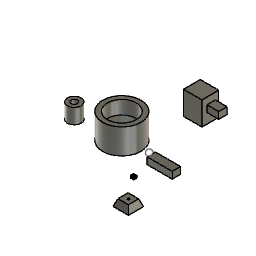
Week 2 Class (Autodesk Fusion 360 design; units mm, degrees)
Autodesk Fusion 360 part; units mm, degrees
sketch "Sketch1" plane through (0, 0, 0) normal (0, 0, 1) x (1, 0, 0)
  line L0 (0, 0) -> (55, 0)
  line L1 (55, 0) -> (55, 50)
  line L2 (55, 50) -> (0, 50)
  line L3 (0, 50) -> (0, 0)
  constraint horizontal L0
  constraint vertical L1
  constraint horizontal L2
  constraint vertical L3
  constraint coincident L0.start L3.end
extrude "Extrude1" add sketch "Sketch1" along normal blind 70 makes body 1
sketch "Sketch2" plane through (55, 0, 0) normal (1, 0, 0) x (0, 1, 0)
  line L0 (0, 0) -> (50, 0)
  line L1 (50, 0) -> (50, 70)
  line L2 (50, 70) -> (0, 70)
  line L3 (0, 70) -> (0, 0)
  line L4 (15, 50) -> (40, 50)
  line L5 (40, 50) -> (40, 30)
  line L6 (40, 30) -> (15, 30)
  line L7 (15, 30) -> (15, 50)
  constraint horizontal L4
  constraint vertical L5
  constraint horizontal L6
  constraint vertical L7
extrude "Extrude2" add sketch "Sketch2" along normal blind 35 contours L4 L5 L6 L7 bodies 1
sketch "Sketch3" plane through (0, 0, 0) normal (0, -1, 0) x (1, 0, 0)
  line L0 (0, 0) -> (55, 0)
  line L1 (55, 0) -> (55, 70)
  line L2 (55, 70) -> (0, 70)
  line L3 (0, 70) -> (0, 0)
sketch "Sketch4" plane through (0, 0, 0) normal (0, 1, 0) x (1, 0, 0)
sketch "Sketch5" plane through (0, 0, 0) normal (0, 1, 0) x (1, 0, 0)
move_body "Move1" bodies 1 to x (1, 0, 0) y (0, 1, 0) z (0, 0, 1) at (0, 35, 0)
sketch "Sketch6" plane through (0, 0, 0) normal (0, 0, 1) x (1, 0, 0)
  circle A0 centre (0, 0) radius 20.4411
  constraint coincident A0.centre origin
extrude "Extrude3" add sketch "Sketch6" along normal blind 45 separate body makes body 2
move_body "Move2" bodies 2 to x (1, 0, 0) y (0, 1, 0) z (0, 0, 1) at (-3.3511, -40.3603, -9.1078)
sketch "Sketch7" plane through (0, 0, 35.8922) normal (0, 0, 1) x (-1, 0, 0)
  circle A0 centre (3.3511, 40.3603) radius 20.4411
  circle A1 centre (3.3511, 40.3603) radius 9.1882
  dimension "d7" = 18.3763
  constraint concentric A0 A1
  measures "d7" diameter of A1
extrude "Extrude4" cut sketch "Sketch7" against normal blind 25 contours A1 bodies 2
extrude "Extrude5" cut 1 faces at (-2.352, -37.8976, 10.8922) along direction (0, 0, -1) blind 129 on bodies 2 bodies 2
move_body "Move3" bodies 2 to x (1, 0, 0) y (0, 1, 0) z (0, 0, 1) at (3.9091, 37.2212, 0)
sketch "Sketch8" plane through (0, 0, 0) normal (1, 0, 0) x (0, 1, 0)
sketch "Sketch9" plane through (0, 0, 0) normal (0, 0, 1) x (1, 0, 0)
sketch "Sketch10" plane through (0, 0, 0) normal (0, 0, 1) x (1, 0, 0)
move_body "Move4" bodies 2 to x (1, 0, 0) y (0, 1, 0) z (0, 0, 1) at (-134.413, -4.3083, 34.1078)
move_body "Move5" bodies 1 to x (1, 0, 0) y (0, 1, 0) z (0, 0, 1) at (64.4102, 84.3152, 34.3939)
sketch "Sketch11" plane through (0, 0, 0) normal (0, 0, 1) x (1, 0, 0)
  circle A0 centre (0, 0) radius 57.0088
  constraint coincident A0.centre origin
extrude "Extrude6" add sketch "Sketch11" along normal blind 75 separate body makes body 3
sketch "Sketch12" plane through (0, 0, 0) normal (0, 0, 1) x (1, 0, 0)
sketch "Sketch13" plane through (0, 0, 75) normal (0, 0, 1) x (-1, 0, 0)
  circle A0 centre (0, 0) radius 57.0088
  circle A1 centre (0, 0) radius 43.0116
  constraint concentric A0 A1
extrude "Extrude7" cut sketch "Sketch13" against normal blind 40 contours A1 bodies 3
sketch "Sketch14" plane through (0, 0, 35) normal (0, 0, 1) x (-1, 0, 0)
  circle A0 centre (0, 0) radius 43.0116
  circle A1 centre (0, 0) radius 11.2283
  constraint coincident A0.centre A1.centre
extrude "Extrude8" cut sketch "Sketch14" against normal blind 90 contours A1 bodies 3
form "Form1" [no effect]
sketch "Sketch15" plane through (0, 0, 0) normal (0, 0, 1) x (1, 0, 0)
  line L0 (100, 0) -> (175, 0)
  line L1 (175, 0) -> (175, -25)
  line L2 (175, -25) -> (100, -25)
  line L3 (100, -25) -> (100, 0)
  constraint horizontal L0
  constraint vertical L1
  constraint horizontal L2
  constraint vertical L3
extrude "Extrude9" add sketch "Sketch15" along normal blind 20 separate body makes body 4
sketch "Sketch16" plane through (0, 0, 20) normal (0, 0, 1) x (-1, 0, 0)
  line L0 (-100, 25) -> (-175, 25)
  line L1 (-175, 25) -> (-175, 0)
  line L2 (-175, 0) -> (-100, 0)
  line L3 (-100, 0) -> (-100, 25)
  line L4 (-58.674, 80.0041, -18.6782) -> (-104.674, 80.0041, -18.6782)
  line L5 (-104.674, 80.0041, -18.6782) -> (-104.674, 125.0041, -18.6782)
  line L6 (-104.674, 125.0041, -18.6782) -> (-58.674, 125.0041, -18.6782)
  line L7 (-58.674, 125.0041, -18.6782) -> (-58.674, 80.0041, -18.6782)
extrude "Extrude10" add sketch "Sketch16" along normal blind 20 draft -20 separate body contours L4 L5 L6 L7 in plane through (0, 0, 1.3218) normal (0, 0, 1) makes body 5
move_face "MoveFace1" by (70, -50, 0) 1 faces at (86.9142, -97.4306, 21.3218) on bodies 5
move_body "Move6" bodies 5 to x (1, 0, 0) y (0, 1, 0) z (0, 0, 1) at (100, -60, 0)
move_body "Move7" bodies 2 to x (1, 0, 0) y (0, 1, 0) z (0, 0, 1) at (1.9174, -2.3531, -31.6058)
sketch "Sketch17" plane through (0, 0, 21.3218) normal (0, 0, 1) x (-1, 0, 0)
  line L0 (-165.9534, 147.2836) -> (-165.9534, 177.7247)
  line L1 (-165.9534, 177.7247) -> (-197.3946, 177.7247)
  line L2 (-197.3946, 177.7247) -> (-197.3946, 147.2836)
  line L3 (-197.3946, 147.2836) -> (-165.9534, 147.2836)
  line L4 (-180, 160) -> (-185, 160)
  line L5 (-185, 160) -> (-185, 165)
  line L6 (-185, 165) -> (-180, 165)
  line L7 (-180, 165) -> (-180, 160)
  constraint horizontal L4
  constraint vertical L5
  constraint horizontal L6
  constraint vertical L7
extrude "Extrude11" cut sketch "Sketch17" against normal blind 110 contours L4 L5 L6 L7 bodies 5
sketch "Sketch18" plane through (0, 0, 0) normal (0, 0, 1) x (1, 0, 0)
  spline S0 degree 3 poles (74.8233, 9.1575) (74.7545, 9.3692) (74.5561, 9.5253) (74.3206, 9.5253) knots 0 0 0 0 1 1 1 1
  line L0 (74.3206, 9.5253) -> (74.056, 9.5253)
  line L1 (74.056, 9.5253) -> (74.056, 10.319)
  arc A0 (73.7914, 10.5836) -> (74.056, 10.319) centre (73.7914, 10.319) cw
  line L2 (73.7914, 10.5836) -> (72.2039, 10.5836)
  line L3 (72.2039, 10.5836) -> (72.2039, 11.1128)
  line L4 (72.2039, 11.1128) -> (72.7331, 11.1128)
  arc A1 (72.9977, 11.3774) -> (72.7331, 11.1128) centre (72.7331, 11.3774) cw
  line L5 (72.9977, 11.3774) -> (72.9977, 11.9065)
  line L6 (72.9977, 11.9065) -> (73.5268, 11.9065)
  arc A2 (74.056, 12.4357) -> (73.5268, 11.9065) centre (73.5268, 12.4357) cw
  line L7 (74.056, 12.4357) -> (74.056, 12.5442)
  spline S1 degree 3 poles (74.056, 12.5442) (74.8312, 12.232) (75.3789, 11.4726) (75.3789, 10.5836) knots 0 0 0 0 1 1 1 1
  spline S2 degree 3 poles (75.3789, 10.5836) (75.3789, 10.0333) (75.1673, 9.5332) (74.8233, 9.1575) knots 0 0 0 0 1 1 1 1
  spline S3 degree 3 poles (72.9977, 8.4855) (71.9526, 8.6151) (71.1456, 9.5041) (71.1456, 10.5836) knots 0 0 0 0 1 1 1 1
  spline S4 degree 3 poles (71.1456, 10.5836) (71.1456, 10.7477) (71.1668, 10.9064) (71.2011, 11.0572) knots 0 0 0 0 1 1 1 1
  line L8 (71.2011, 11.0572) -> (72.4685, 9.7899)
  line L9 (72.4685, 9.7899) -> (72.4685, 9.5253)
  arc A3 (72.9977, 8.9961) -> (72.4685, 9.5253) centre (72.9977, 9.5253) cw
  arc A4 (70.6164, 10.5836) -> (73.2623, 13.2295) centre (73.2623, 10.5836) cw
  arc A5 (73.2623, 7.9378) -> (70.6164, 10.5836) centre (73.2623, 10.5836) cw
  arc A6 (75.9081, 10.5836) -> (73.2623, 7.9378) centre (73.2623, 10.5836) cw
  arc A7 (73.2623, 13.2295) -> (75.9081, 10.5836) centre (73.2623, 10.5836) cw
sketch "Sketch19" plane through (0, 0, 0) normal (0, 0, 1) x (1, 0, 0)
  line L0 (73, 9) -> (73, 8.5)
  constraint vertical L0
sketch "Sketch20" plane through (0, 0, 0) normal (0, 0, 1) x (1, 0, 0)
sketch "Sketch21" plane through (0, 0, 0) normal (0, 0, 1) x (1, 0, 0)
sketch "Sketch22" plane through (0, 0, 0) normal (0, 0, 1) x (1, 0, 0)
sketch "Sketch23" plane through (0, 0, 0) normal (0, 0, 1) x (1, 0, 0)
  line L0 (120, -85) -> (110, -85)
  line L1 (110, -85) -> (110, -75)
  line L2 (110, -75) -> (120, -75)
  line L3 (120, -75) -> (120, -85)
  line L4 (120, -85) -> (110, -75) construction
  line L5 (110, -85) -> (120, -75) construction
  line L6 (117, -82) -> (113, -82)
  line L7 (113, -82) -> (113, -78)
  line L8 (113, -78) -> (117, -78)
  line L9 (117, -78) -> (117, -82)
  line L10 (117, -82) -> (113, -78) construction
  line L11 (113, -82) -> (117, -78) construction
  line L12 (110, -75) -> (113.5, -75)
  line L13 (113.5, -75) -> (113.5, -78.5)
  line L14 (113.5, -78.5) -> (110, -78.5)
  line L15 (110, -78.5) -> (110, -75)
  line L16 (120, -75) -> (116.5, -75)
  line L17 (116.5, -75) -> (116.5, -78.5)
  line L18 (116.5, -78.5) -> (120, -78.5)
  line L19 (120, -78.5) -> (120, -75)
  line L20 (110, -85) -> (113.5, -85)
  line L21 (113.5, -85) -> (113.5, -81.5)
  line L22 (113.5, -81.5) -> (110, -81.5)
  line L23 (110, -81.5) -> (110, -85)
  line L24 (120, -85) -> (116.5, -85)
  line L25 (116.5, -85) -> (116.5, -81.5)
  line L26 (116.5, -81.5) -> (120, -81.5)
  line L27 (120, -81.5) -> (120, -85)
  line L28 (113.5, -78.5) -> (111, -78.5)
  line L29 (111, -78.5) -> (111, -76)
  line L30 (111, -76) -> (113.5, -76)
  line L31 (113.5, -76) -> (113.5, -78.5)
  line L32 (116.5, -78.5) -> (119, -78.5)
  line L33 (119, -78.5) -> (119, -76)
  line L34 (119, -76) -> (116.5, -76)
  line L35 (116.5, -76) -> (116.5, -78.5)
  line L36 (116.5, -81.5) -> (119, -81.5)
  line L37 (119, -81.5) -> (119, -84)
  line L38 (119, -84) -> (116.5, -84)
  line L39 (116.5, -84) -> (116.5, -81.5)
  line L40 (113.5, -81.5) -> (111, -81.5)
  line L41 (111, -81.5) -> (111, -84)
  line L42 (111, -84) -> (113.5, -84)
  line L43 (113.5, -84) -> (113.5, -81.5)
  line L44 (113, -78) -> (114, -78)
  line L45 (117, -78) -> (116, -78)
  line L46 (113, -78) -> (113, -79)
  line L47 (113, -82) -> (113, -81)
  line L48 (113, -82) -> (114, -82)
  line L49 (117, -82) -> (117, -81)
  line L50 (117, -82) -> (116, -82)
  line L51 (114, -78) -> (112, -76)
  line L52 (114, -78) -> (116.8284, -78) construction
  line L53 (113, -79) -> (111, -77)
  line L54 (113, -79) -> (115.8284, -79) construction
  line L55 (113, -81) -> (111, -83)
  line L56 (114, -82) -> (112, -84)
  line L57 (114, -82) -> (116.8284, -82) construction
  line L58 (116, -82) -> (118, -84)
  line L59 (116, -82) -> (118.8284, -82) construction
  line L60 (117, -81) -> (119, -83)
  line L61 (116, -78) -> (118, -76)
  line L62 (116, -78) -> (118.8284, -78) construction
  line L63 (117, -78) -> (117, -79)
  line L64 (117, -79) -> (119, -77)
  line L65 (117, -79) -> (119.8284, -79) construction
  point P0 (115, -80)
  point P1 (115, -80)
  point P2 (115, -80)
  point P3 (115, -80)
  dimension "d33" = 10
  dimension "d34" = 10
  dimension "d43" = 4
  dimension "d44" = 4
  dimension "d45" = 3.5
  dimension "d46" = 3.5
  dimension "d47" = 3.5
  dimension "d48" = 3.5
  dimension "d49" = 3.5
  dimension "d50" = 3.5
  dimension "d51" = 3.5
  dimension "d52" = 3.5
  dimension "d53" = 2.5
  dimension "d54" = 2.5
  dimension "d55" = 2.5
  dimension "d56" = 2.5
  dimension "d57" = 2.5
  dimension "d58" = 2.5
  dimension "d59" = 2.5
  dimension "d60" = 2.5
  dimension "d61" = 1
  dimension "d62" = 1
  dimension "d63" = 1
  dimension "d64" = 1
  dimension "d65" = 1
  dimension "d66" = 1
  dimension "d67" = 1
  dimension "d68" = 135
  dimension "d69" = 135
  dimension "d70" = 90
  dimension "d71" = 135
  dimension "d72" = 45
  dimension "d73" = 180
  dimension "d74" = 45
  dimension "d75" = 1
  dimension "d76" = 45
  constraint horizontal L0
  constraint perpendicular L0 L1
  constraint parallel L0 L2
  constraint parallel L1 L3
  constraint coincident L4 P3
  constraint coincident L5 P3
  constraint coincident P3 P2
  constraint horizontal L6
  constraint perpendicular L6 L7
  constraint parallel L6 L8
  constraint parallel L7 L9
  constraint coincident L10 P3
  constraint coincident L11 P3
  constraint horizontal L12
  constraint vertical L13
  constraint horizontal L14
  constraint vertical L15
  constraint horizontal L16
  constraint vertical L17
  constraint horizontal L18
  constraint vertical L19
  constraint horizontal L20
  constraint vertical L21
  constraint horizontal L22
  constraint vertical L23
  constraint horizontal L24
  constraint vertical L25
  constraint horizontal L26
  constraint vertical L27
  constraint horizontal L28
  constraint vertical L29
  constraint horizontal L30
  constraint vertical L31
  constraint horizontal L32
  constraint vertical L33
  constraint horizontal L34
  constraint vertical L35
  constraint horizontal L36
  constraint vertical L37
  constraint horizontal L38
  constraint vertical L39
  constraint horizontal L40
  constraint vertical L41
  constraint horizontal L42
  constraint vertical L43
  constraint perpendicular L7 L44
  constraint perpendicular L9 L45
  constraint perpendicular L8 L46
  constraint perpendicular L22 L47
  constraint perpendicular L43 L48
  constraint perpendicular L36 L49
  constraint perpendicular L25 L50
  constraint horizontal L52
  constraint coincident L30 L51.end
  constraint horizontal L54
  constraint coincident L29 L53.end
  constraint coincident L41 L55.end
  constraint horizontal L57
  constraint coincident L42 L56.end
  constraint horizontal L59
  constraint coincident L38 L58.end
  constraint coincident L37 L60.end
  constraint horizontal L62
  constraint coincident L34 L61.end
  constraint coincident L9 L63.end
  constraint horizontal L65
  constraint coincident L33 L64.end
  measures "d33" distance of L1.end L2.end
  measures "d34" distance of L0.end L1.end
  measures "d43" distance of L7.end L8.end
  measures "d44" distance of L6.end L7.end
  measures "d45" distance of L1.end L12.end
  measures "d46" distance of L1.end L14.end
  measures "d47" distance of L2.end L16.end
  measures "d48" distance of L2.end L18.end
  measures "d49" distance of L0.end L20.end
  measures "d50" distance of L0.end L22.end
  measures "d51" distance of L0.start L24.end
  measures "d52" distance of L0.start L26.end
  measures "d53" distance of L13.end L28.end
  measures "d54" distance of L13.end L30.end
  measures "d55" distance of L17.end L32.end
  measures "d56" distance of L17.end L34.end
  measures "d57" distance of L25.end L36.end
  measures "d58" distance of L25.end L38.end
  measures "d59" distance of L21.end L40.end
  measures "d60" distance of L21.end L42.end
  measures "d61" distance of L7.end L44.end
  measures "d62" distance of L8.end L45.end
  measures "d63" distance of L7.end L46.end
  measures "d64" distance of L6.end L47.end
  measures "d65" distance of L6.end L48.end
  measures "d66" distance of L6.start L49.end
  measures "d67" distance of L6.start L50.end
  measures "d68" angle of L51 L52
  measures "d69" angle of L53 L54
  measures "d70" angle of L53 L55
  measures "d71" angle of L56 L57
  measures "d72" angle of L58 L59
  measures "d73" angle of L58 L60
  measures "d74" angle of L61 L62
  measures "d75" distance of L8.end L63.end
  measures "d76" angle of L64 L65
extrude "Extrude12" add sketch "Sketch23" along normal blind 7 separate body contours L0 L3 L24 L25 L26 L27 L37 L38 | L0 L1 L20 L21 L22 L23 L41 L42 | L2 L3 L16 L17 L18 L19 L33 L34 | L6 L25 L39 L50 L58 | L6 L9 L25 L26 L36 L37 L38 L39 L49 L50 L58 L60 | L9 L26 L36 L49 L60 | L6 L7 L21 L22 L40 L41 L42 L43 L47 L48 L55 L56 | L6 L21 L43 L48 L56 | L6 L9 L25 L26 L36 L39 L49 L50 | L6 L7 L8 L9 L13 L14 L17 L18 L21 L22 L25 L26 L28 L31 L32 L35 L36 L39 L40 L43 L44 L45 L46 L47 L48 L49 L50 L63 | L9 L18 L32 L63 L64 | L8 L9 L17 L18 L32 L33 L34 L35 L45 L61 L63 L64 | L1 L2 L12 L13 L14 L15 L29 L30 | L6 L7 L21 L22 L40 L43 L47 L48 | L8 L9 L17 L18 L32 L35 L45 L63 | L7 L22 L40 L47 L55 | L8 L17 L35 L45 L61 | L7 L8 L13 L14 L28 L29 L30 L31 L44 L46 L51 L53 | L7 L14 L28 L46 L53 | L8 L13 L31 L44 L51 | L7 L8 L13 L14 L28 L31 L44 L46 makes body 6
sketch "Sketch24" plane through (0, 0, 7) normal (0, 0, 1) x (-1, 0, 0)
  line L0 (-117, 81) -> (-117, 79)
  line L1 (-117, 79) -> (-119, 77)
  line L2 (-119, 77) -> (-119, 78.5)
  line L3 (-119, 78.5) -> (-120, 78.5)
  line L4 (-120, 78.5) -> (-120, 75)
  line L5 (-120, 75) -> (-116.5, 75)
  line L6 (-116.5, 75) -> (-116.5, 76)
  line L7 (-116.5, 76) -> (-118, 76)
  line L8 (-118, 76) -> (-116, 78)
  line L9 (-116, 78) -> (-114, 78)
  line L10 (-114, 78) -> (-112, 76)
  line L11 (-112, 76) -> (-113.5, 76)
  line L12 (-113.5, 76) -> (-113.5, 75)
  line L13 (-113.5, 75) -> (-110, 75)
  line L14 (-110, 75) -> (-110, 78.5)
  line L15 (-110, 78.5) -> (-111, 78.5)
  line L16 (-111, 78.5) -> (-111, 77)
  line L17 (-111, 77) -> (-113, 79)
  line L18 (-113, 79) -> (-113, 81)
  line L19 (-113, 81) -> (-111, 83)
  line L20 (-111, 83) -> (-111, 81.5)
  line L21 (-111, 81.5) -> (-110, 81.5)
  line L22 (-110, 81.5) -> (-110, 85)
  line L23 (-110, 85) -> (-113.5, 85)
  line L24 (-113.5, 85) -> (-113.5, 84)
  line L25 (-113.5, 84) -> (-112, 84)
  line L26 (-112, 84) -> (-114, 82)
  line L27 (-114, 82) -> (-116, 82)
  line L28 (-116, 82) -> (-118, 84)
  line L29 (-118, 84) -> (-116.5, 84)
  line L30 (-116.5, 84) -> (-116.5, 85)
  line L31 (-116.5, 85) -> (-120, 85)
  line L32 (-120, 85) -> (-120, 81.5)
  line L33 (-120, 81.5) -> (-119, 81.5)
  line L34 (-119, 81.5) -> (-119, 83)
  line L35 (-119, 83) -> (-117, 81)
  circle A0 centre (-115, 80) radius 1.25
  dimension "d79" = 2.5
  measures "d79" diameter of A0
extrude "Extrude13" cut sketch "Sketch24" against normal blind 15 contours A0 bodies 6
sketch "Sketch25" plane through (0, 0, 0) normal (0, 0, 1) x (1, 0, 0)
